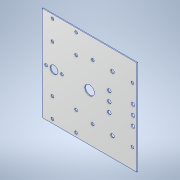
# Autodesk Inventor part: RD002_フレーム
Saved by Autodesk Inventor 2022 (Build 260153000, 153)
## iProperties
Created: 2021-10-14
Part Number: RD002_フレーム
Material: アルミニウム 6061
Document SubType Name: Modeling
Designer: gilte
Density: 2.7 g/cm^3
Appearance: アルミニウム - フラット
Author: gilte
Autodesk Inventor part; units mm, degrees
ref_plane "YZ Plane" through (0, 0, 0) normal (1, 0, 0) x (0, 1, 0)
ref_plane "XZ Plane" through (0, 0, 0) normal (0, 1, 0) x (-1, 0, 0)
ref_plane "XY Plane" through (0, 0, 0) normal (0, 0, 1) x (1, 0, 0)
sketch "スケッチ1" plane through (0, 0, 0) normal (0, 0, 1) x (1, 0, 0)
  line L0 (0, 0) -> (120, 0)
  line L1 (120, 0) -> (120, 120)
  line L2 (120, 120) -> (0, 120)
  line L3 (0, 120) -> (0, 0)
  dimension "d0" = 120
  dimension "d1" = 120
  constraints: 8 end point, 2 parallel, 1 horizontal, 1 perpendicular
  measures "d0" distance of L2.end L1.end
  measures "d1" distance of L1.end L0.end
extrude "押し出し1" add sketch "スケッチ1" along normal blind 1
sketch "スケッチ2" plane through (0, 0, 1) normal (0, 0, 1) x (1, 0, 0)
  line L0 (0, 120) -> (0, 0) projected
  line L1 (0, 60) -> (120, 60)
  line L2 (120, 0) -> (120, 120) projected
  circle A0 centre (60, 60) radius 6
  circle A1 centre (15, 60) radius 5
  circle A2 centre (115, 95.25) radius 1.5
  circle A3 centre (85, 95.25) radius 1.5
  line L3 (120, 120) -> (0, 120) projected
  circle A4 centre (5, 60) radius 1.75
  circle A5 centre (25, 60) radius 1.75
  dimension "d4" = 12
  dimension "d5" = 10
  dimension "d6" = 3
  dimension "d7" = 3
  dimension "d8" = 15
  dimension "d9" = 30
  dimension "d10" = 5
  dimension "d11" = 24.75
  dimension "d12" = 24.75
  dimension "d13" = 3.5
  dimension "d14" = 3.5
  dimension "d15" = 20
  dimension "d16" = 5
  constraints: 6 centre point, 3 midpoint, 3 point on line, 2 end point
  measures "d4" diameter of A0
  measures "d5" diameter of A1
  measures "d6" diameter of A2
  measures "d7" diameter of A3
  measures "d8" distance from line of L0 A1.centre
  measures "d9" distance of A2.centre A3.centre
  measures "d10" distance from line of L2 A2.centre
  measures "d11" distance from line of L3 A2.centre
  measures "d12" distance from line of L3 A3.centre
  measures "d13" diameter of A4
  measures "d14" diameter of A5
  measures "d15" distance of A4.centre A5.centre
  measures "d16" distance from line of L0 A4.centre
extrude "押し出し2" cut sketch "スケッチ2" against normal through all contours A4 L1 | L1 A4 | A0 L1 | L1 A0 | A1 L1 | L1 A1 | A5 L1 | L1 A5 | A2 | A3
sketch "スケッチ3" plane through (0, 0, 1) normal (0, 0, 1) x (1, 0, 0)
  line L0 (0, 120) -> (0, 0) projected
  line L1 (0, 60) -> (120, 60) construction
  line L2 (120, 0) -> (120, 120) projected
  line L3 (120, 120) -> (0, 120) construction
  point P0 (13, 115)
  point P1 (43, 115)
  point P2 (13, 90)
  point P3 (43, 90)
  point P4 (13, 5)
  point P5 (43, 5)
  point P6 (13, 30)
  point P7 (43, 30)
  dimension "d19" = 5
  dimension "d20" = 13
  dimension "d23" = 30
  dimension "d26" = 25
  constraints: 4 symmetric about line, 2 end point, 2 midpoint, 1 horizontal, 1 vertical, 3 other
  measures "d19" distance from line of point (13, 115) L3
  measures "d20" distance from line of L0 point (13, 115)
  measures "d23" distance of point (13, 115) point (43, 115)
  measures "d26" distance of point (13, 115) point (13, 90)
hole "穴1" at (13, 115, 1) at (43, 115, 1) at (13, 90, 1) at (43, 90, 1) at (13, 5, 1) at (43, 5, 1) at (43, 30, 1) at (13, 30, 1) direction (0, 0, -1) diameter 3.5 end through all
sketch "スケッチ4" plane through (0, 0, 1) normal (0, 0, 1) x (1, 0, 0)
  point P0 (0, 0)
sketch "スケッチ5" plane through (0, 0, 1) normal (0, 0, 1) x (1, 0, 0)
  circle A0 centre (85, 95.25) radius 1.5 projected
  circle A1 centre (85, 95.25) radius 1.5
  circle A2 centre (115, 95.25) radius 1.5 projected
  circle A3 centre (115, 95.25) radius 1.5
  point P0 (0, 0)
  constraints: 2 centre point, 2 coincident
extrude "押し出し3" add sketch "スケッチ5" against normal blind 1
sketch "スケッチ6" plane through (0, 0, 1) normal (0, 0, 1) x (1, 0, 0)
  line L0 (0, 120) -> (0, 0) projected
  line L1 (0, 60) -> (120, 60) construction
  line L2 (120, 0) -> (120, 120) projected
  line L3 (0, 0) -> (120, 0) projected
  line L4 (50.2, 60) -> (170.2, 60) construction
  line L5 (120, 120) -> (0, 120) projected
  point P0 (64, 24.75)
  point P1 (114.2, 24.75)
  point P2 (85, 48)
  point P3 (115, 48)
  point P4 (64, 95.25)
  point P5 (114.2, 95.25)
  point P6 (85, 72)
  point P7 (115, 72)
  dimension "d38" = 64
  dimension "d39" = 24.75
  dimension "d42" = 50.2
  dimension "d47" = 72
  dimension "d48" = 85
  dimension "d51" = 30
  constraints: 4 end point, 4 symmetric about line, 2 horizontal, 2 midpoint, 5 other
  measures "d38" distance from line of L0 point (64, 24.75)
  measures "d39" distance from line of L3 point (64, 24.75)
  measures "d42" distance of L1.start L4.start
  measures "d47" distance from line of L5 point (85, 48)
  measures "d48" distance from line of L0 point (85, 48)
  measures "d51" distance of point (85, 48) point (115, 48)
hole "穴2" at (64, 24.75, 1) at (114.2, 24.75, 1) at (85, 48, 1) at (115, 48, 1) at (85, 72, 1) at (115, 72, 1) at (64, 95.25, 1) at (114.2, 95.25, 1) direction (0, 0, -1) diameter 3.5 end through all
sketch "スケッチ7" plane through (0, 0, 1) normal (0, 0, 1) x (1, 0, 0)
  circle A0 centre (85, 72) radius 1.75 projected
  circle A1 centre (85, 72) radius 2.25
  circle A2 centre (115, 72) radius 1.75 projected
  circle A3 centre (115, 72) radius 2.25
  circle A4 centre (115, 48) radius 1.75 projected
  circle A5 centre (115, 48) radius 2.25
  circle A6 centre (85, 48) radius 1.75 projected
  circle A7 centre (85, 48) radius 2.25
  point P0 (0, 0)
  dimension "d63" = 4.5
  dimension "d64" = 4.5
  dimension "d65" = 4.5
  dimension "d66" = 4.5
  constraints: 4 centre point, 4 coincident
  measures "d63" diameter of A1
  measures "d64" diameter of A3
  measures "d65" diameter of A5
  measures "d66" diameter of A7
extrude "押し出し4" cut sketch "スケッチ7" against normal blind 1 contours A0 | A1 | A2 | A3 | A4 | A5 | A6 | A7
sketch "スケッチ9" plane through (0, 0, 1) normal (0, 0, 1) x (1, 0, 0)
  circle A0 centre (85, 72) radius 2.25 construction
  circle A1 centre (85, 48) radius 2.25 construction
  line L0 (85, 72) -> (85, 48) construction
  circle A2 centre (115, 72) radius 2.25 construction
  circle A3 centre (115, 48) radius 2.25 construction
  line L1 (115, 72) -> (115, 48) construction
  point P0 (0, 0)
  point P1 (85, 60)
  point P2 (115, 60)
  constraints: 4 end point, 2 midpoint, 1 parallel, 1 vertical
hole "穴3" at (85, 60, 1) at (115, 60, 1) direction (0, 0, -1) diameter 4.5 depth 1 clearance for "Countersunk Flat Head Screw ISO 2009/7046" size "M4" standard "ISO"
ref_plane "作業平面1" through (0, 60, 0) normal (0, 1, 0) x (1, 0, 0)
sketch "スケッチ10" plane through (0, 0, 1) normal (0, 0, 1) x (1, 0, 0)
  circle A0 centre (64, 95.25) radius 1.75 projected
  circle A1 centre (114.2, 95.25) radius 1.75 projected
  line L0 (64, 95.25) -> (114.2, 95.25)
  circle A2 centre (85, 60) radius 2.25 projected
  circle A3 centre (115, 60) radius 2.25 projected
  line L1 (85, 60) -> (115, 60)
  point P0 (0, 0)
  point P1 (89.1, 95.25)
  point P2 (89.1, 24.75)
  constraints: 4 end point, 2 horizontal, 1 midpoint, 1 symmetric about line
hole "穴4" at (89.1, 95.25, 1) at (89.1, 24.75, 1) direction (0, 0, -1) diameter 4.5 depth 1 clearance for "Countersunk Flat Head Screw ISO 2009/7046" size "M4" standard "ISO"
